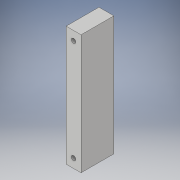
# Autodesk Inventor part: brazo2
Saved by Autodesk Inventor 2019 (Build 230136000, 136)
## iProperties
Created: 2019-10-18
Part Number: brazo2
Material: Genérico
Document SubType Name: Modeling
Designer: Josue
Density: 1 g/cm^3
Appearance: Valor por defecto
Author: Josue
Autodesk Inventor part; units mm, degrees
ref_plane "YZ Plane" through (0, 0, 0) normal (1, 0, 0) x (0, 1, 0)
ref_plane "XZ Plane" through (0, 0, 0) normal (0, 1, 0) x (-1, 0, 0)
ref_plane "XY Plane" through (0, 0, 0) normal (0, 0, 1) x (1, 0, 0)
sketch "Boceto1" plane through (0, 0, 0) normal (0, 1, 0) x (-1, 0, 0)
  line L0 (-25, 55) -> (25, 55)
  line L1 (25, 55) -> (25, -55)
  line L2 (25, -55) -> (-25, -55)
  line L3 (-25, -55) -> (-25, 55)
  line L4 (-25, 55) -> (25, -55) construction
  line L5 (25, 55) -> (-25, -55) construction
  point P0 (0, 0)
  dimension "d0" = 50
  dimension "d1" = 110
  constraints: 12 end point, 2 midpoint, 2 parallel, 1 horizontal, 1 perpendicular
  measures "d0" distance of L1.end L2.end
  measures "d1" distance of L0.end L1.end
extrude "Extrusión1" add sketch "Boceto1" along normal blind 400
sketch "Boceto2" plane through (-25, 0, 55) normal (0, 0, 1) x (1, 0, 0)
  line L0 (0, 400) -> (50, 400) projected
  line L1 (25, 400) -> (25, 370)
  line L2 (25, 0) -> (25, 30)
  circle A0 centre (25, 370) radius 7.5
  circle A1 centre (25, 30) radius 7.5
  dimension "d4" = 30
  dimension "d5" = 30
  dimension "d6" = 15
  dimension "d7" = 15
  constraints: 4 end point, 2 centre point, 2 coincident, 2 vertical, 1 midpoint
  measures "d4" distance of L1.start L1.end
  measures "d5" distance of L2.start L2.end
  measures "d6" diameter of A0
  measures "d7" diameter of A1
extrude "Extrusión2" cut sketch "Boceto2" against normal up to next
